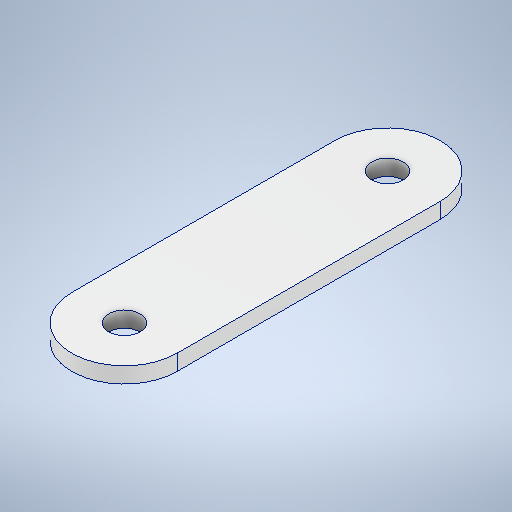
# Autodesk Inventor part: lifter_free_end
Saved by Autodesk Inventor 2025 (Build 290162000, 162)
## iProperties
Created: 2024-04-25
Part Number: lifter_free_end
Material: Hliník 6061
Document SubType Name: Modeling
Designer: rader
Density: 2.7 g/cm^3
Appearance: Hliník – plochý
Author: rader
Autodesk Inventor part; units mm, degrees
ref_plane "YZ Plane" through (0, 0, 0) normal (1, 0, 0) x (0, 1, 0)
ref_plane "XZ Plane" through (0, 0, 0) normal (0, 1, 0) x (-1, 0, 0)
ref_plane "XY Plane" through (0, 0, 0) normal (0, 0, 1) x (1, 0, 0)
sketch "Náčrt1" plane through (0, 0, 0) normal (0, 0, 1) x (1, 0, 0)
  line L0 (0, 17.5) -> (0, 17.5)
  line L1 (5, 12.5) -> (5, -12.5)
  line L2 (0, -17.5) -> (0, -17.5)
  line L3 (-5, -12.5) -> (-5, 12.5)
  line L4 (-8.4497, 0) -> (8.4497, 0) projected
  line L5 (0, 25.9497) -> (0, -25.9497) projected
  arc A0 (0, 17.5) -> (-5, 12.5) centre (0, 12.5) ccw
  arc A1 (5, 12.5) -> (0, 17.5) centre (0, 12.5) ccw
  arc A2 (0, -17.5) -> (5, -12.5) centre (0, -12.5) ccw
  arc A3 (-5, -12.5) -> (0, -17.5) centre (0, -12.5) ccw
  point P0 (0, 0)
  point P1 (-5, 17.5)
  point P2 (5, -17.5)
  point P3 (5, 17.5)
  dimension "d0" = 10
  dimension "d1" = 35
  dimension "d2" = 5
  constraints: 8 end point, 8 point on circle, 8 tangent, 6 point on line, 4 centre point, 3 equal radius, 2 parallel, 1 horizontal, 1 perpendicular, 2 other
  measures "d0" distance of point (-5, 17.5) point (5, 17.5)
  measures "d1" distance of point (5, 17.5) point (5, -17.5)
  measures "d2" radius of A0
extrude "Vysunutí1" add sketch "Náčrt1" along normal mid plane 1.5
sketch "Náčrt2" plane through (0, 0, 0.75) normal (0, 0, 1) x (1, 0, 0)
  arc A0 (-5, -12.5) -> (5, -12.5) centre (0, -12.5) ccw projected
  line L0 (5, -12.5) -> (5, 12.5) projected
  arc A1 (5, 12.5) -> (-5, 12.5) centre (0, 12.5) ccw projected
  line L1 (-5, 12.5) -> (-5, -12.5) projected
  point P0 (0, 0)
  constraints: 2 coincident
hole "Díra1" at (0, 12.5, 0.75) at (0, -12.5, 0.75) direction (0, 0, -1) diameter 3 end through all
